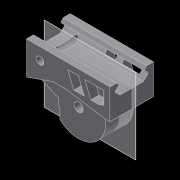
# Autodesk Inventor part: SideHandleBase
Saved by Autodesk Inventor 2020.4 (Build 244396010, 396A)
## iProperties
Created: 2022-09-10
Part Number: SideHandleBase
Material: Generic
Document SubType Name: Modeling
Designer: Val
Density: 1 g/cm^3
Appearance: Default
Author: Val
Autodesk Inventor part; units mm, degrees
ref_plane "YZ Plane" through (0, 0, 0) normal (1, 0, 0) x (0, 1, 0)
ref_plane "XZ Plane" through (0, 0, 0) normal (0, 1, 0) x (-1, 0, 0)
ref_plane "XY Plane" through (0, 0, 0) normal (0, 0, 1) x (1, 0, 0)
sketch "Base" plane through (0, 0, 0) normal (0, 0, 1) x (1, 0, 0)
  line L0 (-12.3981, -13.2027) -> (-12.3981, -7.9395)
  arc A0 (-12.3981, -13.2027) -> (15.9662, 8.5503) centre (0, 0) ccw
  arc A1 (15.9662, 8.5503) -> (5.3507, 16.1838) centre (0.6063, -1.6117) ccw
  arc A2 (5.3507, 16.1838) -> (-4.7343, 14.6301) centre (2.0791, 3.9125) ccw
  arc A3 (-4.7343, 14.6301) -> (-12.3981, -7.9395) centre (5.4695, -1.4207) ccw
  circle A4 centre (0, 0) radius 3
  circle A5 centre (0, 0) radius 3
  circle A6 centre (0, 0) radius 13.497 construction
  line L1 (-28.997, 27.4994) -> (26.303, 27.4994)
  line L2 (4.8764, -0.8461) -> (-14.6101, -0.8461)
  line L3 (-14.6101, -0.8461) -> (-28.997, 5.4994)
  line L4 (-28.997, 5.4994) -> (-28.997, 27.4994)
  line L5 (-28.997, 5.4994) -> (-11.7979, 11.6298)
  line L6 (-11.7979, 11.6298) -> (-2.5387, 11.6298)
  line L7 (-2.5387, 11.6298) -> (23.3778, 7.4994)
  line L8 (23.3778, 7.4994) -> (26.303, 7.4994)
  line L9 (26.303, 27.4994) -> (26.303, 7.4994)
  line L10 (4.8764, -0.8461) -> (26.303, 7.4994)
  line L11 (22.303, 23.4994) -> (9.7408, 23.4994)
  line L12 (9.7408, 23.4994) -> (13.5825, 13.7045)
  line L13 (13.5825, 13.7045) -> (19.1614, 13.7045)
  line L14 (19.1614, 13.7045) -> (22.303, 14.9367)
  line L15 (22.303, 14.9367) -> (22.303, 23.4994)
  line L16 (5.4441, 23.4994) -> (-1.5148, 23.4994)
  line L17 (-1.5148, 23.4994) -> (2.3269, 13.7045)
  line L18 (2.3269, 13.7045) -> (9.2858, 13.7045)
  line L19 (9.2858, 13.7045) -> (5.4441, 23.4994)
  circle A7 centre (-19.997, 19.4307) radius 2.5
  arc A8 (-4.7343, 14.6301) -> (-12.3981, -7.9395) centre (5.4695, -1.4207) ccw
  line L20 (-13.497, 0) -> (-13.497, -16.2978) construction
  point P0 (11.7017, -28.7626)
  point P1 (-13.5415, -0.8461)
  point P2 (15.8686, 8.6961)
  point P3 (-2.8782, -0.8461)
  point P4 (2.8782, -0.8461)
  point P5 (17.6358, 4.1236)
  dimension "d0" = 22
  dimension "d1" = 20
  dimension "d2" = 5
  dimension "d3" = 9
  dimension "d4" = 4
  dimension "d5" = 4
  dimension "d6" = 4
  dimension "d7" = 55.3
  dimension "d8" = 15.5
  constraints: 42 end point, 11 point on circle, 8 centre point, 6 parallel, 4 horizontal, 3 perpendicular, 2 vertical, 1 coincident, 1 collinear, 1 horizontal alignment, 2 other
  measures "d0" distance of L4.start L4.end
  measures "d1" distance of L1.end L10.end
  measures "d2" diameter of A7
  measures "d3" distance from line of L4 A7.centre
  measures "d4" distance between parallel lines of L1 L16
  measures "d5" distance between parallel lines of L12 L19
  measures "d6" distance between parallel lines of L9 L15
  measures "d7" distance of L4.end L1.end
  measures "d8" distance between parallel lines of L4 L20
extrude "BaseFeature" add sketch "Base" along normal blind 18.2 contours L0 A3 L2 A4 L10 A0 | L10 L2 A4 A3 L6 L7 A1 A0 | L2 L3 L5 L6 A3 | L8 L7 A1 L19 L16 L17 A2 A3 L6 L5 L4 L1 L9 | A3 A2 L17 L18 L19 A1 L7 L6 | L19 L18 L17 A2 A1 | A1 A2 L17 L16 L19 | L15 L14 L13 L12 L11
extrude "ExtendFeature" add sketch "Base" along normal blind 23.72 contours L8 L7 A1 L19 L16 L17 A2 A3 L6 L5 L4 L1 L9 | A3 A2 L17 L18 L19 A1 L7 L6
extrude "Extend2Feature" add sketch "Base" against normal blind 5.2 contours L8 L7 A1 L19 L16 L17 A2 A3 L6 L5 L4 L1 L9 | A3 A2 L17 L18 L19 A1 L7 L6
sketch "PicatinnyRail" plane through (-28.997, 5.4994, 23.72) normal (-1, 0, 0) x (0, 0, 1)
  line L0 (-23.72, 0) -> (-5.52, 0) projected
  line L1 (-5.52, 0) -> (0, 0) projected
  line L2 (0, 22) -> (0, 0) projected
  line L3 (-28.92, 22) -> (0, 22) construction
  line L4 (-28.92, 0) -> (-28.92, 22) projected
  line L5 (-23.72, 0) -> (-28.92, 0) projected
  line L6 (-22.21, 14) -> (-6.71, 14)
  line L7 (-14.46, 14) -> (-14.46, 22) construction
  line L8 (-28.92, 22) -> (0, 22) construction
  line L9 (-28.92, 22) -> (0, 22) construction
  line L10 (-6.71, 14) -> (-3.71, 14) construction
  line L11 (0, 18) -> (0, 8.2052) projected
  line L12 (-22.21, 14) -> (-25.21, 14) construction
  line L13 (-3.71, 14) -> (-3.71, 17) construction
  line L14 (-25.21, 14) -> (-25.21, 17) construction
  line L15 (-23.72, 18) -> (-28.92, 18) projected
  line L16 (-6.71, 14) -> (-3.71, 17)
  line L17 (-22.21, 14) -> (-25.21, 17)
  line L18 (-3.71, 17) -> (-25.21, 17) construction
  line L19 (-3.71, 17) -> (-3.71, 18)
  line L20 (-25.21, 17) -> (-25.21, 18)
  line L21 (-3.71, 18) -> (-6.21, 20)
  line L22 (-3.71, 18) -> (-3.71, 20) construction
  line L23 (-3.71, 20) -> (-6.21, 20) construction
  line L24 (-6.21, 20) -> (-4.61, 22)
  line L25 (-25.21, 18) -> (-22.71, 20)
  line L26 (-22.71, 20) -> (-24.31, 22)
  line L27 (-24.31, 22) -> (-4.61, 22)
  point P0 (-23.72, -5.4994)
  dimension "d15" = 15.5
  dimension "d16" = 3
  dimension "d17" = 3
  dimension "d18" = 3
  dimension "d19" = 1
  dimension "d20" = 2
  dimension "d21" = 2.5
  dimension "d22" = 2
  dimension "d23" = 38.66
  dimension "d24" = 38.66
  constraints: 36 end point, 5 perpendicular, 4 equal length, 3 horizontal, 3 vertical, 2 midpoint, 2 point on line, 1 collinear
  measures "d15" distance of L6.start L6.end
  measures "d16" distance of L6.end L10.end
  measures "d17" distance of L10.end L13.end
  measures "d18" distance of L12.end L14.end
  measures "d19" distance of L13.end L19.end
  measures "d20" distance of L19.end L22.end
  measures "d21" distance of L22.end L21.end
  measures "d22" vertical distance of L21.end L24.end
  measures "d23" angle of L21 L18
  measures "d24" angle of L18 L25
extrude "PicatinnyRailCut" cut sketch "PicatinnyRail" against normal through all
ref_plane "MidPlane" through (0, 0, 9.26) normal (0, 0, 1) x (1, 0, 0)
equation "\"d24\" = d23"
body "Solid1"
